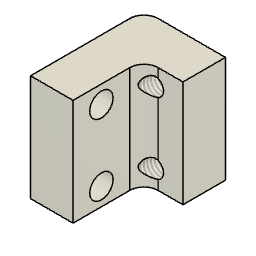
escuadra_bluetooth_bracket_v5 (Autodesk Fusion 360 design; units mm, degrees)
Autodesk Fusion 360 part; units mm, degrees
sketch "Sketch1" plane through (0, 0, 0) normal (0, 0, 1) x (1, 0, 0)
  line L0 (7.5, 7.5) -> (-7.5, 7.5)
  line L1 (-7.5, 7.5) -> (-7.5, -7.5)
  line L2 (-7.5, -7.5) -> (7.5, -7.5)
  line L3 (7.5, -7.5) -> (7.5, 7.5)
  line L4 (7.5, 7.5) -> (-7.5, -7.5) construction
  line L5 (-7.5, 7.5) -> (7.5, -7.5) construction
  line L6 (0, -7.5) -> (0, 7.5) construction
  circle A0 centre (0, 5) radius 1.5
  line L7 (0, 0) -> (7.5, 0) construction
  circle A1 centre (0, -5) radius 1.5
  line L8 (-7.5, 7.5) -> (-4.5, 7.5)
  line L9 (-4.5, 7.5) -> (-4.5, -7.5)
  line L10 (-4.5, -7.5) -> (-7.5, -7.5)
  line L11 (-7.5, -7.5) -> (-7.5, 7.5)
  line L12 (4, -7.5) -> (4, 7.5)
  dimension "d1" = 3
  dimension "d2" = 5
  dimension "d3" = 15
  dimension "d4" = 15
  dimension "d7" = 3
  dimension "d20" = 4
  constraint horizontal L0
  constraint perpendicular L0 L1
  constraint parallel L0 L2
  constraint parallel L1 L3
  constraint coincident L4 L7.start
  constraint coincident L5 L7.start
  constraint coincident L7.start origin
  constraint midpoint L2 L6.start
  constraint midpoint L0 L6.end
  constraint coincident L6 A0.centre
  constraint midpoint L3 L7.end
  constraint symmetric A0 L7 A1
  constraint horizontal L8
  constraint vertical L9
  constraint horizontal L10
  constraint vertical L11
  constraint coincident L2 L9.end
  constraint coincident L2 L12.start
  constraint coincident L0 L12.end
  constraint perpendicular L0 L12
  measures "d1" diameter of A0
  measures "d2" distance of L7.start A0.centre
  measures "d3" distance of L0.start L2
  measures "d4" distance of L1.end L2.end
  measures "d7" distance of L1 L9
  measures "d20" distance of A0.centre L12
extrude "Extrude1" add sketch "Sketch1" against normal blind 3 contours L0 L2 L9 L12 | L0 L1 L2 L8 L9 L10 L11
extrude "Extrude2" add sketch "Sketch1" along normal blind 13 contours L0 L1 L2 L8 L9 L10 L11
sketch "Sketch2" plane through (-7.5, 0, 0) normal (-1, 0, 0) x (0, 0, 1)
  line L0 (13, 7.5) -> (-3, 7.5)
  line L1 (-3, 7.5) -> (-3, -7.5)
  line L2 (-3, -7.5) -> (13, -7.5)
  line L3 (13, -7.5) -> (13, 7.5)
  line L4 (-3, 0) -> (9, 0) construction
  line L5 (9, 0) -> (9, 5) construction
  circle A0 centre (9, 5) radius 1.65
  circle A1 centre (9, -5) radius 1.65
  dimension "d11" = 12
  dimension "d16" = 3.3
  dimension "d17" = 5
  constraint midpoint L1 L4.start
  constraint perpendicular L1 L4
  constraint perpendicular L4 L5
  constraint coincident L5.end A0.centre
  constraint symmetric L4 A0 A1
  measures "d11" distance of L4.start L4.end
  measures "d16" diameter of A0
  measures "d17" distance of L4.end L5.end
extrude "Extrude3" cut sketch "Sketch2" against normal blind 3 contours A0 | A1
fillet "Fillet1" radius 2 2 edges at (-4.5, 0, 0) (-7.5, 0, -3)
thread "Thread1" "ISO Metric profile 3.0 M3x0.5 6H" major diameter 3.086 minor diameter 2.529 pitch 0.5 angle 60 resizes the face on face at (1.4981, -5.0748, -2) on face at (1.4981, 4.9252, -2)
move_face "OffsetFaces1" offset 3 1 faces at (-4.5, 1.3568, 3.8789)
move_face "OffsetFaces2" offset 3 1 faces at (3.0187, 1.4349, 0)
